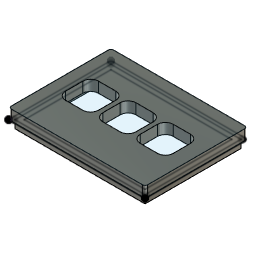
Button Case Lid (Autodesk Fusion 360 design; units mm, degrees)
Autodesk Fusion 360 part; units mm, degrees
sketch "Sketch1" plane through (0, 0, 0) normal (0, 0, 1) x (1, 0, 0)
  line L0 (1, 0) -> (51, 0)
  line L1 (52, 1) -> (52, 38)
  line L2 (51, 39) -> (1, 39)
  line L3 (0, 38) -> (0, 1)
  arc A0 (1, 39) -> (0, 38) centre (1, 38) ccw
  arc A1 (52, 38) -> (51, 39) centre (51, 38) ccw
  arc A2 (51, 0) -> (52, 1) centre (51, 1) ccw
  arc A3 (0, 1) -> (1, 0) centre (1, 1) ccw
  line L4 (1.2, 37.8) -> (1.2, 1.2)
  line L5 (1.2, 1.2) -> (50.8, 1.2)
  line L6 (50.8, 1.2) -> (50.8, 37.8)
  line L7 (50.8, 37.8) -> (1.2, 37.8)
  line L8 (49, 3) -> (49, 36)
  line L9 (49, 36) -> (3, 36)
  line L10 (3, 36) -> (3, 3)
  line L11 (3, 3) -> (49, 3)
  point P0 (52, 0)
  point P1 (0, 39)
  dimension "d1" = 52
  dimension "d2" = 39
  dimension "d3" = 1
  dimension "d6" = -1.2
  dimension "d7" = -3
  constraint horizontal L0
  constraint vertical L1
  constraint horizontal L2
  constraint vertical L3
  constraint coincident P1 L2
  constraint coincident P1 L3
  constraint tangent L2 A0
  constraint tangent L3 A0
  constraint tangent L1 A1
  constraint tangent L2 A1
  constraint equal A0 A1
  constraint coincident P0 L0
  constraint coincident P0 L1
  constraint tangent L0 A2
  constraint tangent L1 A2
  constraint equal A0 A2
  constraint coincident origin L0
  constraint coincident origin L3
  constraint tangent L0 A3
  constraint tangent L3 A3
  constraint equal A0 A3
  measures "d1" distance of origin P0
  measures "d2" distance of origin P1
  measures "d3" radius of A0
extrude "Extrude1" add sketch "Sketch1" along normal blind 4 contours L0 L1 L2 L3 A0 A1 A2 A3 | L4 L5 L6 L7 | L8 L9 L10 L11
sketch "Sketch2" plane through (0, 0, 4) normal (0, 0, 1) x (-1, 0, 0)
  arc A0 (0, -1) -> (-1, 0) centre (-1, -1) ccw
  line L0 (-1, 0) -> (-51, 0)
  arc A1 (-51, 0) -> (-52, -1) centre (-51, -1) ccw
  line L1 (-52, -1) -> (-52, -38)
  arc A2 (-52, -38) -> (-51, -39) centre (-51, -38) ccw
  line L2 (-51, -39) -> (-1, -39)
  arc A3 (-1, -39) -> (0, -38) centre (-1, -38) ccw
  line L3 (0, -38) -> (0, -1)
sketch "Sketch3" plane through (0, 0, 4) normal (0, 0, 1) x (-1, 0, 0)
extrude "Extrude2" add sketch "Sketch1" against normal blind 3 contours L4 L5 L6 L7
sketch "Sketch4" plane through (0, 0, 4) normal (0, 0, 1) x (-1, 0, 0)
sketch "Sketch5" plane through (0, 0, 4) normal (0, 0, 1) x (-1, 0, 0)
  line L0 (-43.5, -13.25) -> (-36.9, -13.25)
  line L1 (-33.9, -16.25) -> (-33.9, -22.85)
  line L2 (-36.9, -25.85) -> (-43.5, -25.85)
  line L3 (-46.5, -22.85) -> (-46.5, -16.25)
  arc A0 (-43.5, -13.25) -> (-46.5, -16.25) centre (-43.5, -16.25) ccw
  arc A1 (-33.9, -16.25) -> (-36.9, -13.25) centre (-36.9, -16.25) ccw
  arc A2 (-36.9, -25.85) -> (-33.9, -22.85) centre (-36.9, -22.85) ccw
  arc A3 (-46.5, -22.85) -> (-43.5, -25.85) centre (-43.5, -22.85) ccw
  line L4 (-1, 0) -> (-51, 0)
  line L5 (-49, -3) -> (-49, -36)
  line L6 (-29.25, -13.25) -> (-22.65, -13.25)
  arc A4 (-29.25, -13.25) -> (-32.25, -16.25) centre (-29.25, -16.25) ccw
  line L7 (-32.25, -22.85) -> (-32.25, -16.25)
  arc A5 (-32.25, -22.85) -> (-29.25, -25.85) centre (-29.25, -22.85) ccw
  arc A6 (-22.65, -25.85) -> (-19.65, -22.85) centre (-22.65, -22.85) ccw
  line L8 (-22.65, -25.85) -> (-29.25, -25.85)
  line L9 (-19.65, -16.25) -> (-19.65, -22.85)
  arc A7 (-19.65, -16.25) -> (-22.65, -13.25) centre (-22.65, -16.25) ccw
  line L10 (-15, -13.25) -> (-8.4, -13.25)
  arc A8 (-15, -13.25) -> (-18, -16.25) centre (-15, -16.25) ccw
  line L11 (-18, -22.85) -> (-18, -16.25)
  arc A9 (-18, -22.85) -> (-15, -25.85) centre (-15, -22.85) ccw
  arc A10 (-8.4, -25.85) -> (-5.4, -22.85) centre (-8.4, -22.85) ccw
  line L12 (-8.4, -25.85) -> (-15, -25.85)
  line L13 (-5.4, -16.25) -> (-5.4, -22.85)
  arc A11 (-5.4, -16.25) -> (-8.4, -13.25) centre (-8.4, -16.25) ccw
  point P0 (-46.5, -13.25)
  point P1 (-33.9, -13.25)
  point P2 (-46.5, -25.85)
  dimension "d10" = 12.6
  dimension "d11" = 12.6
  dimension "d12" = 3
  dimension "d13" = 13.25
  dimension "d14" = 2.5
  dimension "d17" = 14.25
  dimension "d18" = 0
  constraint horizontal L0
  constraint vertical L1
  constraint horizontal L2
  constraint vertical L3
  constraint coincident P0 L0
  constraint coincident P0 L3
  constraint tangent L0 A0
  constraint tangent L3 A0
  constraint coincident P1 L0
  constraint coincident P1 L1
  constraint tangent L0 A1
  constraint tangent L1 A1
  constraint equal A0 A1
  constraint tangent L1 A2
  constraint tangent L2 A2
  constraint equal A0 A2
  constraint coincident P2 L2
  constraint coincident P2 L3
  constraint tangent L2 A3
  constraint tangent L3 A3
  constraint equal A0 A3
  measures "d10" distance of P0 P1
  measures "d11" distance of P0 P2
  measures "d12" radius of A0
  measures "d13" distance of L0 L4
  measures "d14" distance of L3 L5
extrude "Extrude3" cut sketch "Sketch5" against normal blind 8
